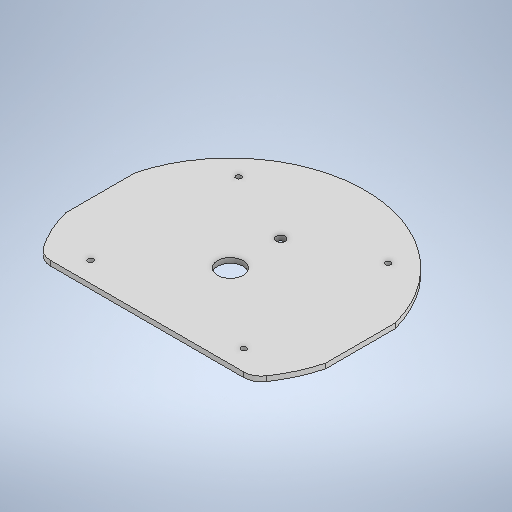
# Autodesk Inventor part: tapa_carcasa_4.0_v2
Saved by Autodesk Inventor 2025.3 (Build 293356030, 356C)
## iProperties
Created: 2025-11-26
Part Number: tapa_carcasa_4.0_v2
Material: Generic
Document SubType Name: Modeling
Designer: brene
Density: 1 g/cm^3
Appearance: Default
Author: brene
Autodesk Inventor part; units mm, degrees
ref_plane "YZ Plane" through (0, 0, 0) normal (1, 0, 0) x (0, 1, 0)
ref_plane "XZ Plane" through (0, 0, 0) normal (0, 1, 0) x (-1, 0, 0)
ref_plane "XY Plane" through (0, 0, 0) normal (0, 0, 1) x (1, 0, 0)
sketch "Sketch1" plane through (0, 0, 0) normal (0, 1, 0) x (-1, 0, 0)
  line L0 (0, 0) -> (71, 0)
  line L1 (71, 0) -> (71, -19.0066)
  line L2 (71, 0) -> (71, 19.0066)
  line L3 (0, 0) -> (0, -73.5)
  line L4 (-71, 0) -> (-71, -19.0066)
  line L5 (-71, 0) -> (-71, 19.0066)
  line L6 (0, 0) -> (0, 45.5)
  line L7 (0, 45.5) -> (52.6498, 45.5)
  line L8 (0, 45.5) -> (-52.6498, 45.5)
  arc A0 (-60.9411, 41.0906) -> (-71, 19.0066) centre (0, 0) ccw
  arc A1 (-71, -19.0066) -> (71, -19.0066) centre (0, 0) ccw
  arc A2 (71, 19.0066) -> (60.9411, 41.0906) centre (0, 0) ccw
  arc A3 (60.9411, 41.0906) -> (52.6498, 45.5) centre (52.6498, 35.5) ccw
  arc A4 (-52.6498, 45.5) -> (-60.9411, 41.0906) centre (-52.6498, 35.5) ccw
  point P0 (57.7235, 45.5)
  point P1 (-57.7235, 45.5)
  dimension "d62" = 71
  dimension "d63" = 45.5
  dimension "d64" = 10
  constraints: 18 end point, 13 point on circle, 5 centre point, 4 tangent, 2 perpendicular, 2 point on line, 2 vertical, 1 equal radius, 1 horizontal, 1 symmetric about line
  measures "d62" distance of L0.start L0.end
  measures "d63" distance of L0.start L6.end
  measures "d64" radius of A3
extrude "Extrusion1" add sketch "Sketch1" along normal blind 2.7
sketch "Sketch2" plane through (0, 2.7, 0) normal (0, 1, 0) x (1, 0, 0)
  circle A0 centre (0, 0) radius 7
  line L0 (0, 0) -> (0, 73.5)
  line L1 (0, 73.5) -> (0, 27.5)
  circle A1 centre (0, 27.5) radius 2.5
  circle A2 centre (0, 0) radius 54.1913 construction
  line L2 (0, 0) -> (-67.8888, -56.0453) construction
  line L3 (0, 0) -> (-54.1913, 0)
  circle A3 centre (-41.7906, -34.5) radius 1.5
  circle A4 centre (41.7906, -34.5) radius 1.5
  circle A5 centre (0, 0) radius 61 construction
  line L4 (0, 0) -> (-40.817, 45.3318)
  circle A6 centre (-40.817, 45.3318) radius 1.5
  circle A7 centre (40.817, 45.3318) radius 1.5
  circle A8 centre (0, 0) radius 73.5 construction
  dimension "d48" = 122
  dimension "d38" = 14
  dimension "d39" = 46
  dimension "d40" = 5
  dimension "d41" = 108.3827
  dimension "d42" = 39.541
  dimension "d43" = 3
  dimension "d47" = 67.8888
  dimension "d50" = 48
  dimension "d52" = 3
  constraints: 10 end point, 7 centre point, 5 coincident, 2 point on circle, 2 point on line, 2 symmetric about line, 1 horizontal, 1 vertical, 1 vertical alignment, 7 other
  measures "d38" diameter of A0
  measures "d39" distance of L0.end L1.end
  measures "d40" diameter of A1
  measures "d41" diameter of A2
  measures "d42" angle of L3 L2
  measures "d43" diameter of A3
  measures "d47" distance from line of L2.end L0
  measures "d50" angle of L3 L4
  measures "d52" diameter of A6
extrude "Extrusion2" cut sketch "Sketch2" against normal blind 2.7
body "Solid1"
